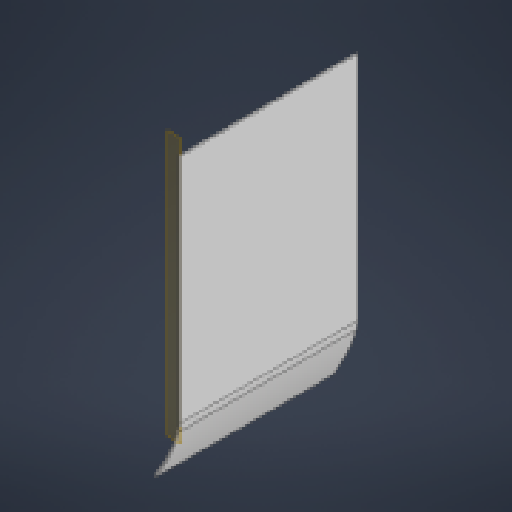
# Autodesk Inventor part: Intake main polycarb
Saved by Autodesk Inventor 2023 (Build 270158000, 158)
## iProperties
Created: 2023-03-22
Part Number: Intake main polycarb
Material: Generic
Document SubType Name: Modeling
Designer: Main Account
Density: 1 g/cm^3
Appearance: Default
Author: Main Account
Autodesk Inventor part; units mm, degrees
ref_plane "YZ Plane" through (0, 0, 0) normal (1, 0, 0) x (0, 1, 0)
ref_plane "XZ Plane" through (0, 0, 0) normal (0, 1, 0) x (-1, 0, 0)
ref_plane "XY Plane" through (0, 0, 0) normal (0, 0, 1) x (1, 0, 0)
ref_plane "Work Plane1" through (0, 0, 0) normal (0, 0, 1) x (1, 0, 0)
sketch "Sketch1" plane through (0, 0, 0) normal (0, 0, 1) x (1, 0, 0)
  line L0 (-5.0952, -133.1293) -> (-4.7767, -132.9202) construction
  arc A0 (-5.0952, -133.1293) -> (-0.7466, -139.7544) centre (-1.0882, -135.2389) ccw construction
  line L1 (4.7811, 106.7831) -> (4.7811, -102.6288)
  arc A1 (-17.4789, -155.8337) -> (3.6681, -110.0654) centre (-174.5174, -55.5054) ccw
  line L2 (4.7811, 106.7831) -> (3.1936, 106.7831)
  line L3 (4.7811, -105.9343) -> (6.3686, -105.9343) construction
  line L4 (3.1936, -102.5821) -> (3.1936, 106.7831)
  line L5 (-17.4789, -155.8337) -> (-18.8167, -154.979)
  line L6 (-174.5174, -55.5054) -> (-175.8552, -54.6508)
  line L7 (-174.5174, -55.5054) -> (-172.9299, -55.5054) construction
  arc A2 (-18.8167, -154.979) -> (2.0412, -110.1462) centre (-175.8552, -54.6508) ccw
  line L8 (3.1936, -105.9343) -> (3.1936, -105.9468)
  arc A3 (2.0412, -110.1462) -> (3.1936, -102.5821) centre (-22.2064, -102.5821) ccw
  arc A4 (3.6681, -110.0654) -> (4.7811, -102.6288) centre (-20.6189, -102.6288) ccw
  point P0 (0, 0)
  point P1 (4.7811, -106.2883)
  dimension "d1" = 1.5875
  dimension "d6" = 1.5875
  dimension "d7" = 1.5875
  dimension "d8" = 147.426
  dimension "d13" = 25.4
  constraints: 18 end point, 11 point on circle, 5 centre point, 5 tangent, 4 point on line, 3 coincident, 3 horizontal, 2 vertical, 1 equal length, 1 equal radius, 1 line through centre, 8 other
  measures "d1" distance of L1.start L2.end
  measures "d6" distance of L5.end L5.start
  measures "d7" distance of L6.start L6.end
  measures "d8" angle of L7 L6
  measures "d13" radius of A3
extrude "Extrusion1" add sketch "Sketch1" against normal blind 158.75
body "Solid1"
